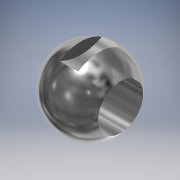
# Autodesk Inventor part: Ball
Saved by Autodesk Inventor 2018 (Build 220112000, 112)
## iProperties
Shininess: 64.0
Length Units: 11269
Angle Units: 11279
Time Units: 11290
Mass Units: 11283
Length Display Precision: 3
Angle Display Precision: 2
Compacted: True
Part Number: Ball
Document SubType Name: Modeling
Created: 2003-04-24
Designer: James M. Leake
Material: Stainless Steel, 440C
Density: 7.75 g/cm^3
Appearance: Semi-Polished
Density: 0.0
Volumn: 0.0
Area: 0.0
PropertySet Name: Model Information
Control State: 0
Master: False
Checked Out: False
Author: James M. Leake
Autodesk Inventor part; units mm, degrees
ref_plane "YZ Plane" through (0, 0, 0) normal (1, 0, 0) x (0, 1, 0)
ref_plane "XZ Plane" through (0, 0, 0) normal (0, 1, 0) x (-1, 0, 0)
ref_plane "XY Plane" through (0, 0, 0) normal (0, 0, 1) x (1, 0, 0)
sketch "Sketch1" plane through (0, 0, 0) normal (0, 0, 1) x (1, 0, 0)
  line L0 (-2.7, 0) -> (35.1, 0) projected
  line L1 (0, -32.4) -> (0, 43.2) projected
  arc A0 (0, -27) -> (0, 27) centre (0, 0) ccw
  line L2 (0, -27) -> (0, 27)
  dimension "d0" = 54
  constraints: 2 end point, 2 point on circle, 1 centre point, 1 coincident, 1 collinear, 1 point on line
  measures "d0" diameter of A0
revolve "Revolution1" add sketch "Sketch1" angle 360 about axis through (0, -10, 0) along (0, 1, 0)
sketch "Sketch2" plane through (0, 0, 0) normal (1, 0, 0) x (0, 1, 0)
  line L0 (-38.4, 0) -> (51.2, 0) projected
  line L1 (0, -37.9) -> (0, 114.7) projected
  circle A0 centre (0, 0) radius 16
  circle A1 centre (0, 0) radius 27 projected
  circle A2 centre (0, 50) radius 32
  dimension "d2" = 32
  dimension "d5" = 32
  dimension "d6" = 50
  constraints: 2 centre point, 1 coincident, 1 point on line
  measures "d2" diameter of A0
  measures "d5" radius of A2
  measures "d6" distance from line of L0 A2.centre
extrude "Extrusion1" cut sketch "Sketch2" along normal through all both and the other way through all contours A0 L1 L0 | L0 L1 A0 | L1 A0 L0 | L0 A0 L1
extrude "Extrusion2" cut sketch "Sketch2" against normal mid plane 13 contours A2 L1 A1 | A1 L1 A2 | A2 A1 L1 | A1 A2 L1
body "Solid1"
